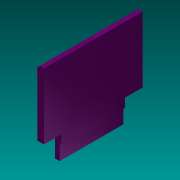
# Autodesk Inventor part: MotorClipV3Front
Saved by Autodesk Inventor 2013 (Build 170138000, 138)
## iProperties
Created: 2013-08-16
Part Number: MotorClipV3Front
Material: ABS Plastic
Document SubType Name: Modeling
Designer: Sawaiz
Density: 1 g/cm^3
Author: Sawaiz
Autodesk Inventor part; units mm, degrees
ref_plane "YZ Plane" through (0, 0, 0) normal (1, 0, 0) x (0, 1, 0)
ref_plane "XZ Plane" through (0, 0, 0) normal (0, 1, 0) x (-1, 0, 0)
ref_plane "XY Plane" through (0, 0, 0) normal (0, 0, 1) x (1, 0, 0)
sketch "Sketch1" plane through (0, 0, 0) normal (1, 0, 0) x (0, 1, 0)
  line L0 (-1.5, 6.858) -> (1.5, 6.858)
  line L1 (1.5, 6.858) -> (1.5, -6.858)
  line L2 (1.5, -6.858) -> (-1.5, -6.858)
  line L3 (-1.5, -6.858) -> (-1.5, 6.858)
  line L4 (-1.5, 6.858) -> (1.5, -6.858) construction
  line L5 (1.5, 6.858) -> (-1.5, -6.858) construction
  line L6 (1.5, 6.858) -> (39.5, 6.858)
  line L7 (39.5, 6.858) -> (39.5, 9.858)
  line L8 (39.5, 9.858) -> (1.5, 9.858)
  line L9 (1.5, 9.858) -> (1.5, 6.858)
  line L10 (1.5, -6.858) -> (39.5, -6.858)
  line L11 (39.5, -6.858) -> (39.5, -9.858)
  line L12 (39.5, -9.858) -> (1.5, -9.858)
  line L13 (1.5, -9.858) -> (1.5, -6.858)
  line L14 (9.5, 6.858) -> (1.5, 6.858)
  line L15 (1.5, 6.858) -> (1.5, -0.142)
  line L16 (1.5, -0.142) -> (9.5, -0.142)
  line L17 (9.5, -0.142) -> (9.5, 6.858)
  line L18 (9.5, -6.858) -> (1.5, -6.858)
  line L19 (1.5, -6.858) -> (1.5, -0.142)
  line L20 (1.5, -0.142) -> (9.5, -0.142)
  line L21 (9.5, -0.142) -> (9.5, -6.858)
  line L22 (9.5, -0.142) -> (1.5, -0.142)
  line L23 (1.5, 6.858) -> (-1.5, 6.858)
  line L24 (-1.5, 6.858) -> (-1.5, 9.858)
  line L25 (-1.5, 9.858) -> (1.5, 9.858)
  line L26 (1.5, 9.858) -> (1.5, 6.858)
  line L27 (1.5, -6.858) -> (-1.5, -6.858)
  line L28 (-1.5, -6.858) -> (-1.5, -9.858)
  line L29 (-1.5, -9.858) -> (1.5, -9.858)
  line L30 (1.5, -9.858) -> (1.5, -6.858)
  point P0 (0, 0)
  dimension "d0" = 3
  dimension "d2" = 13.716
  dimension "d3" = 3
  dimension "d4" = 3
  dimension "d5" = 38
  dimension "d6" = 38
  dimension "d7" = 0
  dimension "d8" = 8
  dimension "d9" = 8
  dimension "d12" = 7
  dimension "d13" = 6.716
  constraints: 62 end point, 14 parallel, 8 perpendicular, 7 horizontal, 4 point on line, 2 midpoint
  measures "d0" distance of L1.end L2.end
  measures "d2" distance of L0.end L1.end
  measures "d3" distance of L6.end L7.end
  measures "d4" distance of L10.end L11.end
  measures "d5" distance of L11.end L12.end
  measures "d6" distance of L7.end L8.end
  measures "d7" distance between parallel lines of L1 L15
  measures "d8" distance between parallel lines of L15 L17
  measures "d9" distance between parallel lines of L19 L21
  measures "d12" distance between parallel lines of L6 L22
  measures "d13" distance between parallel lines of L18 L16
extrude "Extrusion1" add sketch "Sketch1" along normal blind 45
sketch "Sketch2" plane through (0, -1.5, 9.858) normal (0, 0, 1) x (1, 0, 0)
  line L0 (5, 7) -> (8.9446, 7) projected
  arc A0 (5, 7) -> (5, 0) centre (5, 3.5) ccw projected
  line L1 (8.9446, 0) -> (5, 0) projected
  arc A1 (13.3822, 14.1239) -> (31.6178, 14.1239) centre (22.5, 3.5) ccw projected
  line L2 (13.3822, 14.1239) -> (13.3822, 15.7096) projected
  line L3 (13.6751, 16.4167) -> (15.15, 17.8916) projected
  arc A2 (13.6751, 16.4167) -> (13.3822, 15.7096) centre (14.3822, 15.7096) ccw projected
  arc A3 (16.15, 20.3916) -> (15.15, 19.3916) centre (16.15, 19.3916) ccw projected
  line L4 (15.15, 19.3916) -> (15.15, 17.8916) projected
  line L5 (28.85, 20.3916) -> (16.15, 20.3916) projected
  arc A4 (29.85, 19.3916) -> (28.85, 20.3916) centre (28.85, 19.3916) ccw projected
  line L6 (29.85, 17.8916) -> (29.85, 19.3916) projected
  line L7 (31.3249, 16.4167) -> (29.85, 17.8916) projected
  line L8 (31.6178, 15.7096) -> (31.6178, 14.1239) projected
  arc A5 (31.6178, 15.7096) -> (31.3249, 16.4167) centre (30.6178, 15.7096) ccw projected
  line L9 (40, 7) -> (36.0554, 7) projected
  arc A6 (40, 0) -> (40, 7) centre (40, 3.5) ccw projected
  line L10 (36.0554, 0) -> (40, 0) projected
  line L11 (40, 7) -> (36.0554, 7) projected
  arc A7 (40, 0) -> (40, 7) centre (40, 3.5) ccw projected
  line L12 (36.0554, 0) -> (40, 0) projected
  line L13 (8.9446, 0) -> (5, 0) projected
  line L14 (36.0554, 0) -> (40, 0) projected
  line L15 (0, 41) -> (0, 0) projected
  line L16 (0, 0) -> (45, 0) projected
  line L17 (45, 41) -> (45, 0) projected
  line L18 (0, 41) -> (45, 41) projected
  line L19 (5, 7) -> (8.9446, 7) projected
  arc A8 (5, 7) -> (5, 0) centre (5, 3.5) ccw projected
sketch "Sketch3" plane through (0, -1.5, 9.858) normal (0, 0, 1) x (1, 0, 0)
  line L0 (0, 0) -> (45, 0) projected
  line L1 (45, 41) -> (45, 0) projected
  point P0 (0, 41)
  point P1 (0, 1.5)
  point P2 (5, 3.5)
  point P3 (40, 3.5)
  dimension "d16" = 35
  dimension "d18" = 5
  dimension "d19" = 45
  dimension "d20" = 3.5
  dimension "d21" = 3.5
  measures "d16" distance of point (40, 3.5) point (5, 3.5)
  measures "d18" distance from line of L1 point (40, 3.5)
  measures "d19" distance of point (0, 41) L1.start
  measures "d20" distance from line of L0 point (5, 3.5)
  measures "d21" distance from line of L0 point (40, 3.5)
hole "Hole1" at (5, 2, 9.858) at (40, 2, 9.858) direction (0, 0, -1) diameter 4.2 end through all
extrude "Extrusion2" cut sketch "Sketch2" against normal blind 0.82 contours A1 L2 A2 L3 L4 A3 L5 A4 L6 L7 A5 L8 L16 | L16 A1
sketch "Sketch4" plane through (0, -1.5, 9.858) normal (0, 0, 1) x (1, 0, 0)
  arc A0 (36.0554, 0) -> (31.6178, 14.1239) centre (22.5, 3.5) ccw projected
  line L0 (36.0554, 0) -> (45, 0) projected
  arc A1 (13.3822, 14.1239) -> (8.9446, 0) centre (22.5, 3.5) ccw projected
  circle A2 centre (5, 3.5) radius 2.1 projected
  circle A3 centre (40, 3.5) radius 2.1 projected
  arc A4 (5, 7) -> (5, 0) centre (5, 3.5) ccw projected
  line L1 (5, 7) -> (8.9446, 7) projected
  line L2 (8.9446, 0) -> (5, 0) projected
  arc A5 (13.3822, 14.1239) -> (31.6178, 14.1239) centre (22.5, 3.5) ccw projected
  arc A6 (13.3822, 14.1239) -> (31.6178, 14.1239) centre (22.5, 3.5) ccw projected
  line L3 (40, 7) -> (36.0554, 7) projected
  arc A7 (40, 0) -> (40, 7) centre (40, 3.5) ccw projected
  line L4 (36.0554, 0) -> (40, 0) projected
  point P0 (0, 1.5)
extrude "Extrusion3" cut sketch "Sketch4" against normal blind 0.82
sketch "Sketch5" plane through (0, -1.5, -9.858) normal (0, 0, -1) x (-1, 0, 0)
  circle A0 centre (-5, 3.5) radius 2.1 projected
  circle A1 centre (-40, 3.5) radius 2.1 projected
  line L0 (-34.959, 3.5) -> (-37.4795, -0.8656)
  line L1 (-37.4795, -0.8656) -> (-42.5205, -0.8656)
  line L2 (-42.5205, -0.8656) -> (-45.041, 3.5)
  line L3 (-45.041, 3.5) -> (-42.5205, 7.8656)
  line L4 (-42.5205, 7.8656) -> (-37.4795, 7.8656)
  line L5 (-37.4795, 7.8656) -> (-34.959, 3.5)
  line L6 (0.041, 3.5) -> (-2.4795, -0.8656)
  line L7 (-2.4795, -0.8656) -> (-7.5205, -0.8656)
  line L8 (-7.5205, -0.8656) -> (-10.041, 3.5)
  line L9 (-10.041, 3.5) -> (-7.5205, 7.8656)
  line L10 (-7.5205, 7.8656) -> (-2.4795, 7.8656)
  line L11 (-2.4795, 7.8656) -> (0.041, 3.5)
  point P0 (0, 1.5)
  point P1 (-40, 3.5)
  point P2 (-5, 3.5)
  dimension "d33" = 8.7312
  dimension "d34" = 8.7312
  constraints: 24 end point, 2 coincident, 26 other
  measures "d33" distance between parallel lines of L1 L4
  measures "d34" distance between parallel lines of L7 L10
extrude "Extrusion4" cut sketch "Sketch5" against normal blind 3.175
sketch "Sketch6" plane through (0, 9.5, 6.858) normal (0, 1, 0) x (1, 0, 0)
  line L0 (7.5, 1.82) -> (37.5, 1.82) projected
  line L1 (37.5, 9.82) -> (7.5, 9.82) projected
  line L2 (7.5, 1.82) -> (7.5, 9.82)
  line L3 (37.5, 1.82) -> (37.5, 9.82)
  line L4 (7, 10.32) -> (38, 10.32)
  line L5 (38, 10.32) -> (38, 1.32)
  line L6 (38, 1.32) -> (7, 1.32)
  line L7 (7, 1.32) -> (7, 10.32)
  line L8 (8, 10.32) -> (37, 10.32)
  line L9 (37, 10.32) -> (37, 1.32)
  line L10 (37, 1.32) -> (8, 1.32)
  line L11 (8, 1.32) -> (8, 10.32)
  line L12 (0, 0) -> (45, 0) projected
  line L13 (8, 1.32) -> (37, 1.32)
  line L14 (37, 1.32) -> (37, 0)
  line L15 (37, 0) -> (8, 0)
  line L16 (8, 0) -> (8, 1.32)
  point P0 (0, 6.858)
  dimension "d37" = 0.5
  dimension "d56" = 1
  dimension "d57" = 1
  constraints: 28 end point, 6 parallel, 4 perpendicular, 3 point on line, 2 horizontal, 3 other
  measures "d37" distance between parallel lines of L1 L4
  measures "d56" distance between parallel lines of L5 L9
  measures "d57" distance between parallel lines of L7 L11
chamfer "Chamfer1" distance 1 angle 45 2 edges at (22.5, 39.5, -6.858) (22.5, 39.5, 6.858)
sketch "Sketch7" plane through (0, 9.5, -6.858) normal (0, 0, 1) x (1, 0, 0)
  line L0 (0, 29) -> (0, 0) projected
  line L1 (0, 0) -> (45, 0) projected
  line L2 (45, 29) -> (45, 0) projected
  circle A0 centre (22.5, 10) radius 4.318
  line L3 (22.5, 10) -> (22.5, 20)
  circle A1 centre (22.5, 20) radius 2.159
  line L4 (20.341, 20) -> (20.341, 6.2605)
  line L5 (24.659, 20) -> (24.659, 6.2605)
  point P0 (0, -9.5)
  dimension "d43" = 8.636
  dimension "d45" = 10
  dimension "d46" = 4.318
  dimension "d47" = 22.5
  dimension "d48" = 45
  dimension "d49" = 10
  constraints: 6 end point, 4 point on circle, 3 parallel, 2 centre point, 2 tangent, 1 coincident
  measures "d43" diameter of A0
  measures "d45" distance of L3.start L3.end
  measures "d46" diameter of A1
  measures "d47" distance from line of L0 L3.start
  measures "d48" distance of L0.end L1.end
  measures "d49" distance from line of L1 L3.start
extrude "Extrusion6" cut sketch "Sketch7" against normal through all
sketch "Sketch8" plane through (0, 9.5, -6.858) normal (0, 0, 1) x (1, 0, 0)
  arc A0 (20.341, 13.7395) -> (24.659, 13.7395) centre (22.5, 10) ccw projected
  line L0 (20.341, 13.7395) -> (20.341, 20) projected
  arc A1 (24.659, 20) -> (20.341, 20) centre (22.5, 20) ccw projected
  line L1 (24.659, 20) -> (24.659, 13.7395) projected
  line L2 (45, 29) -> (45, 0) projected
  circle A2 centre (22.5, 20) radius 4.318
  line L3 (18.182, 20) -> (18.182, 10)
  line L4 (26.818, 10) -> (26.818, 20)
  point P0 (0, -9.5)
  dimension "d52" = 4.318
  dimension "d53" = 8.636
  constraints: 4 end point, 4 point on circle, 2 parallel, 2 tangent, 1 centre point, 1 coincident
  measures "d52" radius of A0
  measures "d53" diameter of A2
extrude "Extrusion7" cut sketch "Sketch8" against normal blind 2 contours L0 A2 L1 A0 | A0 L3 A2 L0 | A2 L1 A1 L0 | A0 L1 A2 L4 picked at (24.9024, 17.6839)
extrude "Extrusion8" cut sketch "Sketch6" against normal through all contours L11 L1 L9 L0 | L0 L9 L6 L11 | L6 L14 L12 L16 | L11 L4 L9 L1
sketch "Sketch9" plane through (0, 0, 0) normal (-1, 0, 0) x (0, 0, 1)
  line L0 (-30, 50) -> (6.858, 50)
  line L1 (6.858, 50) -> (6.858, -18)
  line L2 (6.858, -18) -> (-30, -18)
  line L3 (-30, -18) -> (-30, 50)
  point P0 (0, 0)
  constraints: 8 end point, 2 parallel, 1 horizontal, 1 perpendicular
extrude "Extrusion9" cut sketch "Sketch9" against normal through all
sketch "Sketch10" plane through (0, -1.5, 9.858) normal (0, 0, 1) x (1, 0, 0)
  line L0 (8, 11) -> (0, 11)
  line L1 (0, 11) -> (0, 0)
  line L2 (0, 0) -> (8, 0)
  line L3 (8, 0) -> (8, 11)
  line L4 (37, 11) -> (45, 11)
  line L5 (45, 11) -> (45, 0)
  line L6 (45, 0) -> (37, 0)
  line L7 (37, 0) -> (37, 11)
  point P0 (0, 1.5)
  constraints: 16 end point, 4 parallel, 2 horizontal, 2 perpendicular, 2 other
extrude "Extrusion10" cut sketch "Sketch10" against normal through all
equation "\"d2\" = StretcherDepth"
equation "\"d6\" = d5"
equation "\"d9\" = d8"
equation "\"d18\" = -0.5 * d16 + 0.5 * d19"
equation "\"d47\" = 0.5 * d48"
equation "\"d53\" = 2 * d52"
equation "\"StretcherDepth\" = 13.716"
body "Solid1"
